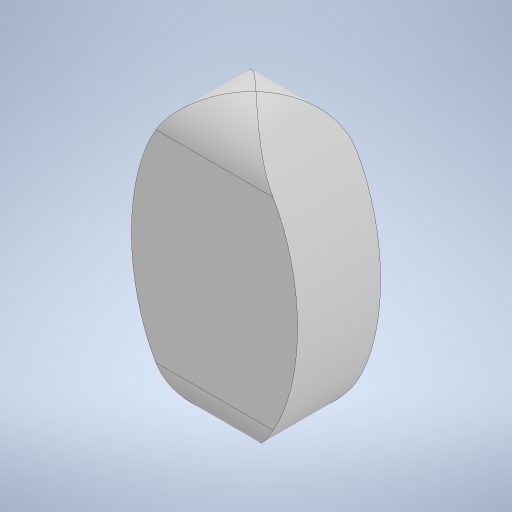
# Autodesk Inventor part: bloqueador2XD
Saved by Autodesk Inventor 2024.4 (Build 284460000, 460)
## iProperties
Created: 2026-06-02
Part Number: bloqueador2XD
Material: Generic
Document SubType Name: Modeling
Designer: Apleppli
Density: 1 g/cm^3
Appearance: Default
Author: Apleppli
Autodesk Inventor part; units mm, degrees
ref_plane "YZ Plane" through (0, 0, 0) normal (1, 0, 0) x (0, 1, 0)
ref_plane "XZ Plane" through (0, 0, 0) normal (0, 1, 0) x (-1, 0, 0)
ref_plane "XY Plane" through (0, 0, 0) normal (0, 0, 1) x (1, 0, 0)
sketch "Sketch1" plane through (0, 0, 0) normal (0, 0, 1) x (1, 0, 0)
  line L0 (5.7625, -8) -> (-5.7625, -8)
  line L1 (-5.7625, -8) -> (-5.7625, 8)
  line L2 (-5.7625, 8) -> (5.7625, 8)
  line L3 (5.7625, 8) -> (5.7625, -8)
  line L4 (5.7625, -8) -> (-5.7625, 8) construction
  line L5 (-5.7625, -8) -> (5.7625, 8) construction
  line L6 (0, 8) -> (0, -8)
  line L7 (0, 8) -> (0, 19.7625)
  line L8 (0, -8) -> (0, -4.35)
  ellipse E0 centre (0, 0) end of major axis (0, 19.7625) minor radius 11.525
  point P0 (0, -8)
  dimension "d4" = 11.525
  dimension "d7" = 19.7625
  dimension "diametro" = 11.525
  dimension "altura" = 16
  dimension "d2" = 5.7625
  constraints: 18 end point, 4 midpoint, 3 coincident, 2 parallel, 2 vertical, 1 horizontal, 1 perpendicular, 1 point on line, 1 vertical alignment, 2 other
  measures "diametro" distance of L1.end L2.end
  measures "altura" distance of L0.end L1.end
  measures "d2" distance between parallel lines of L6 L1
extrude "Extrusion1" add sketch "Sketch1" along normal mid plane 11.525 contours L0 L6 L2 L3 | L0 L1 L2 L6 | E0
sketch "Sketch2" plane through (0, 0, 0) normal (1, 0, 0) x (0, 1, 0)
  line L0 (-19.7625, -5.7625) -> (19.7625, -5.7625) projected
  line L1 (19.7625, 5.7625) -> (-19.7625, 5.7625) projected
  line L2 (-14, -5.7625) -> (14, -5.7625)
  line L3 (14, -5.7625) -> (14, 5.7625)
  line L4 (14, 5.7625) -> (-14, 5.7625)
  line L5 (-14, 5.7625) -> (-14, -5.7625)
  line L6 (-14, -5.7625) -> (14, 5.7625) construction
  line L7 (14, -5.7625) -> (-14, 5.7625) construction
  line L8 (0, 0) -> (14, 0)
  circle A0 centre (14, 0) radius 5.7625
  circle A1 centre (-14, 0) radius 5.7625
  line L9 (14, 0) -> (19.7625, 0)
  line L10 (-14, 0) -> (-19.7625, 0)
  line L11 (-19.7625, 5.7625) -> (-19.7625, -5.7625)
  line L12 (19.7625, 5.7625) -> (19.7625, -5.7625)
  point P0 (17.8, 4.8)
  point P1 (-17.8, 4.8)
  point P2 (17.8, 0)
  point P3 (17.8, -4.8)
  point P4 (17.8, 4.8)
  point P5 (-17.8, -4.8)
  point P6 (8.2375, 0)
  point P7 (-17.8, 4.8)
  dimension "d8" = 28
  constraints: 22 end point, 4 midpoint, 4 point on circle, 2 centre point, 2 horizontal, 2 parallel, 2 perpendicular, 2 point on line, 1 coincident, 1 vertical
  measures "d8" distance of L4.end L3.end
extrude "Extrusion2" cut sketch "Sketch2" along normal mid plane 60 contours A1 L1 A0 L0 | A1 L10 L5 | L5 A1 | A1 L5 L10 | A0 L8 L3 | L3 L9 A0 | L8 A0 L3 | L3 A0 L9 keep common part
sketch "Sketch10" plane through (0.6119, -2.6811, 15.2375) normal (0, 0, -1) x (-0.8342492, -0.5513875, 0)
  line L0 (-3.4624, 1.4166) -> (-3.3124, 1.4279) projected
  line L1 (-3.3124, 1.4279) -> (-3.3651, 1.5156) projected
  line L2 (-3.3651, 1.5156) -> (-3.4624, 1.4166) projected
  line L3 (-3.0104, 0.7328) -> (-2.8606, 0.7916) projected
  arc A0 (-2.9364, 0.8757) -> (-2.8606, 0.7916) centre (-0.9678, 2.5741) ccw projected
  line L4 (-2.9364, 0.8757) -> (-3.0104, 0.7328) projected
  line L5 (-2.3769, 0.2125) -> (-2.2511, 0.3128) projected
  arc A1 (-2.3483, 0.3709) -> (-2.2511, 0.3128) centre (-0.9678, 2.5741) ccw projected
  line L6 (-2.3483, 0.3709) -> (-2.3769, 0.2125) projected
  line L7 (-1.6182, -0.0979) -> (-1.5276, 0.035) projected
  arc A2 (-1.6376, 0.0618) -> (-1.5276, 0.035) centre (-0.9678, 2.5741) ccw projected
  line L8 (-1.6376, 0.0618) -> (-1.6182, -0.0979) projected
  line L9 (-0.8017, -0.1709) -> (-0.7543, -0.0171) projected
  arc A3 (-0.8673, -0.024) -> (-0.7543, -0.0171) centre (-0.9678, 2.5741) ccw projected
  line L10 (-0.8673, -0.024) -> (-0.8017, -0.1709) projected
  line L11 (0, 0) -> (0, 0.1609) projected
  arc A4 (-0.106, 0.1211) -> (0, 0.1609) centre (-0.9678, 2.5741) ccw projected
  line L12 (-0.106, 0.1211) -> (0, 0) projected
  line L13 (0.7157, 0.3996) -> (0.6683, 0.5534) projected
  arc A5 (0.5787, 0.484) -> (0.6683, 0.5534) centre (-0.9678, 2.5741) ccw projected
  line L14 (0.5787, 0.484) -> (0.7157, 0.3996) projected
  line L15 (1.2819, 0.9925) -> (1.1912, 1.1254) projected
  arc A6 (1.1261, 1.0328) -> (1.1912, 1.1254) centre (-0.9678, 2.5741) ccw projected
  line L16 (1.1261, 1.0328) -> (1.2819, 0.9925) projected
  line L17 (1.6481, 1.7258) -> (1.5223, 1.8261) projected
  arc A7 (1.4874, 1.7184) -> (1.5223, 1.8261) centre (-0.9678, 2.5741) ccw projected
  line L18 (1.4874, 1.7184) -> (1.6481, 1.7258) projected
  line L19 (1.7819, 2.5346) -> (1.6321, 2.5933) projected
  arc A8 (1.6305, 2.4801) -> (1.6321, 2.5933) centre (-0.9678, 2.5741) ccw projected
  line L20 (1.6305, 2.4801) -> (1.7819, 2.5346) projected
  line L21 (1.5428, 3.2501) -> (1.6714, 3.3468) projected
  line L22 (1.6714, 3.3468) -> (1.5109, 3.3588) projected
  arc A9 (1.5428, 3.2501) -> (1.5109, 3.3588) centre (-0.9678, 2.5741) ccw projected
  arc A10 (1.232, 3.9601) -> (1.1695, 4.0546) centre (-0.9678, 2.5741) ccw projected
  line L23 (1.232, 3.9601) -> (1.3264, 4.0904) projected
  line L24 (1.3264, 4.0904) -> (1.1695, 4.0546) projected
  line L25 (0.7775, 4.6993) -> (0.7252, 4.669) projected
  line L26 (0.7252, 4.669) -> (0.7538, 4.6295) projected
  line L27 (0.7538, 4.6295) -> (0.7775, 4.6993) projected
  point P0 (-0.9678, 2.5741)
sketch "Sketch13" plane through (0, 14, 19.45) normal (0, 0, -1) x (-1, 0, 0)
  line L0 (1.9982, 0.0857) -> (2.507, -11.7764) projected
  line L1 (2.0018, 0) -> (2.507, -11.7764) projected
  arc A0 (1.9982, 0.0857) -> (-1.9982, 0.0857) centre (0, 0) ccw projected
  line L2 (2.507, -16.2236) -> (2.0018, -28) projected
  line L3 (2.507, -16.2236) -> (1.9982, -28.0857) projected
  arc A1 (-1.9982, -28.0857) -> (1.9982, -28.0857) centre (0, -28) ccw projected
  arc A2 (2.507, -11.7764) -> (2.5354, -11.8489) centre (2.6269, -11.7712) ccw projected
  arc A3 (2.507, -11.7764) -> (2.5354, -11.8489) centre (2.6269, -11.7712) ccw projected
  arc A4 (2.5354, -16.1511) -> (2.507, -16.2236) centre (2.6269, -16.2288) ccw projected
  arc A5 (2.5354, -16.1511) -> (2.507, -16.2236) centre (2.6269, -16.2288) ccw projected
  line L4 (-2.507, -11.7764) -> (-1.9982, 0.0857) projected
  line L5 (-2.507, -11.7764) -> (-2.0018, 0) projected
  line L6 (-2.0018, -28) -> (-2.507, -16.2236) projected
  line L7 (-1.9982, -28.0857) -> (-2.507, -16.2236) projected
  arc A6 (-2.5354, -11.8489) -> (-2.507, -11.7764) centre (-2.6269, -11.7712) ccw projected
  arc A7 (-2.5354, -11.8489) -> (-2.507, -11.7764) centre (-2.6269, -11.7712) ccw projected
  arc A8 (-2.507, -16.2236) -> (-2.5354, -16.1511) centre (-2.6269, -16.2288) ccw projected
  arc A9 (-2.507, -16.2236) -> (-2.5354, -16.1511) centre (-2.6269, -16.2288) ccw projected
  circle A10 centre (0, -14) radius 1.375 projected
  circle A11 centre (0, -14) radius 1.375 projected
  circle A12 centre (0, -14) radius 3.325
  circle A13 centre (0, -14) radius 2.275 projected
  circle A14 centre (0, -14) radius 1.375 projected
  line L8 (-1.9982, -28.0857) -> (-2.0018, -28) projected
  line L9 (-2.0018, 0) -> (-1.9982, 0.0857) projected
  line L10 (2.0018, -28) -> (1.9982, -28.0857) projected
  line L11 (1.9982, 0.0857) -> (2.0018, 0) projected
  point P0 (0, -14)
  point P1 (2.5354, -11.8489)
  point P2 (1.9982, 0.0857)
  point P3 (1.7327, 0.9988)
  point P4 (-2.5354, -11.8489)
  point P5 (-2.5354, -16.1511)
  point P6 (-1.9982, -28.0857)
  point P7 (-1.7327, -28.9988)
  point P8 (2.5354, -16.1511)
  point P9 (1.9982, -28.0857)
  point P10 (1.9982, 0.0857)
  point P11 (-1.9982, 0.0857)
  constraints: 1 centre point, 1 coincident, 2 other
sketch "Sketch14" plane through (0, 0, 19.45) normal (0, 0, -1) x (-1, 0, 0)
  circle A0 centre (0, 0) radius 2.275 projected
  point P0 (0, 0)
sketch "Sketch15" plane through (6.3413, 14, 15.2375) normal (0, 0, -1) x (-1, 0, 0)
  circle A0 centre (6.3413, -14) radius 4
  dimension "d43" = 8
  constraints: 1 centre point, 1 coincident
  measures "d43" diameter of A0
sketch "Sketch3" plane through (0, 0, 1.45) normal (0, 0, 1) x (1, 0, 0)
  circle A0 centre (0, 0) radius 2.275 projected
  circle A1 centre (0, 0) radius 1.375 projected
sketch "Sketch5" plane through (0, 0, -2.2) normal (0, 0, -1) x (-1, 0, 0)
  arc A0 (-2.5354, 2.1511) -> (-2.5354, -2.1511) centre (0, 0) ccw
  arc A1 (-2.5027, 2.1891) -> (-2.5354, 2.1511) centre (0, 0) ccw
  arc A2 (2.2925, 2.4083) -> (-2.2925, 2.4083) centre (0, 0) ccw
  arc A3 (2.5354, 2.1511) -> (2.5027, 2.1891) centre (0, 0) ccw
  arc A4 (2.5354, -2.1511) -> (2.5354, 2.1511) centre (0, 0) ccw
  arc A5 (2.5027, -2.1891) -> (2.5354, -2.1511) centre (0, 0) ccw
  arc A6 (-2.2925, -2.4083) -> (2.2925, -2.4083) centre (0, 0) ccw
  arc A7 (-2.5354, -2.1511) -> (-2.5027, -2.1891) centre (0, 0) ccw
  circle A8 centre (0, 0) radius 3.325
  line L0 (-1.9982, 14.0857) -> (-2.507, 2.2236)
  arc A9 (-2.5354, 2.1511) -> (-2.507, 2.2236) centre (-2.6269, 2.2288) ccw
  arc A10 (2.5354, 2.1511) -> (-2.5354, 2.1511) centre (0, 0) ccw
  arc A11 (2.507, 2.2236) -> (2.5354, 2.1511) centre (2.6269, 2.2288) ccw
  line L1 (2.507, 2.2236) -> (1.9982, 14.0857)
  arc A12 (1.9982, 14.0857) -> (-1.9982, 14.0857) centre (0, 14) ccw
  arc A13 (-2.507, -2.2236) -> (-2.5354, -2.1511) centre (-2.6269, -2.2288) ccw
  line L2 (-2.507, -2.2236) -> (-1.9982, -14.0857)
  arc A14 (-1.9982, -14.0857) -> (1.9982, -14.0857) centre (0, -14) ccw
  line L3 (1.9982, -14.0857) -> (2.507, -2.2236)
  arc A15 (2.5354, -2.1511) -> (2.507, -2.2236) centre (2.6269, -2.2288) ccw
  arc A16 (-2.5354, -2.1511) -> (2.5354, -2.1511) centre (0, 0) ccw
  spline S0 degree 3 poles (-2.5027, 2.1891) (-2.4878, 2.2061) (-2.4695, 2.2267) (-2.4037, 2.2984) (-2.3494, 2.3542) (-2.2925, 2.4083) knots 0 0 0 0 0.303042 0.303042 1 1 1 1
  spline S1 degree 3 poles (2.2925, 2.4083) (2.3494, 2.3541) (2.4036, 2.2985) (2.4693, 2.2269) (2.4878, 2.2061) (2.5027, 2.1891) knots 0 0 0 0 0.696524 0.696524 1 1 1 1
  spline S2 degree 3 poles (2.5027, -2.1891) (2.4878, -2.2061) (2.4695, -2.2267) (2.4037, -2.2984) (2.3494, -2.3542) (2.2925, -2.4083) knots 0 0 0 0 0.303042 0.303042 1 1 1 1
  spline S3 degree 3 poles (-2.2925, -2.4083) (-2.3494, -2.3541) (-2.4036, -2.2985) (-2.4693, -2.2269) (-2.4878, -2.2061) (-2.5027, -2.1891) knots 0 0 0 0 0.696524 0.696524 1 1 1 1
equation "\"d4\" = diametro"
equation "\"d2\" = 0.5 * diametro"
equation "\"d5\" = diametro"
body "Solid2"
body "Solid1"
